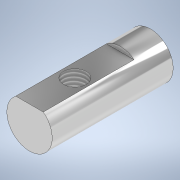
# Autodesk Inventor part: motor shaft
Saved by Autodesk Inventor 2020 (Build 240168000, 168)
## iProperties
Created: 2020-07-28
Part Number: motor shaft
Material: Steel, Mild
Document SubType Name: Modeling
Designer: Ashiqrahman
Density: 7.85 g/cm^3
Appearance: Chrome - Polished
Mass: 3.11402 g
Surface Area: 3.89334 cm^2
Volume: 0.39669 cm^3
Author: Ashiqrahman
Autodesk Inventor part; units mm, degrees
ref_plane "YZ Plane" through (0, 0, 0) normal (1, 0, 0) x (0, 1, 0)
ref_plane "XZ Plane" through (0, 0, 0) normal (0, 1, 0) x (-1, 0, 0)
ref_plane "XY Plane" through (0, 0, 0) normal (0, 0, 1) x (1, 0, 0)
sketch "Sketch1" plane through (0, 0, 0) normal (0, 0, 1) x (1, 0, 0)
  circle A0 centre (0, 0) radius 3 projected
  circle A1 centre (0, 0) radius 5 projected
  dimension "d0" = 10
  dimension "d1" = 6
  measures "d0" diameter of A1
  measures "d1" diameter of A0
extrude "Extrusion1" add sketch "Sketch1" along normal blind 16 contours A0
sketch "Sketch2" plane through (0, 0, 16) normal (0, 0, 1) x (1, 0, 0)
  circle A0 centre (0, 0) radius 3 projected
  line L0 (-1.8209, 2.3842) -> (1.8209, 2.3842)
  line L1 (-3, 0) -> (3, 0)
  constraints: 4 end point, 4 point on circle, 2 horizontal, 1 parallel
extrude "Extrusion2" cut sketch "Sketch2" against normal blind 12 contours L0 A0
sketch "Sketch3" plane through (-1.8209, 2.3842, 16) normal (0, 1, 0) x (1, 0, 0)
  circle A0 centre (1.8209, 6) radius 1.5
  line L0 (3.6417, 0) -> (0, 0) projected
  point P0 (1.8209, 16)
  dimension "d6" = 6
  dimension "d7" = 3
  constraints: 1 centre point
  measures "d6" distance from line of A0.centre L0
  measures "d7" diameter of A0
extrude "Extrusion3" cut sketch "Sketch3" against normal up to surface
thread "Thread1" size "M3x0.5" class "6H" standard "ANSI Metric M Profile" length 60
body "Solid1"
